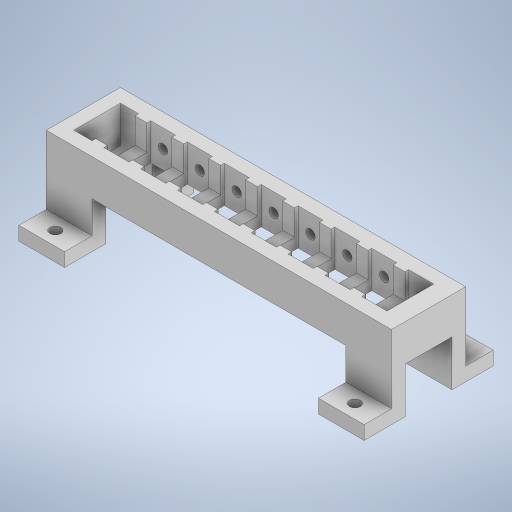
# Autodesk Inventor part: LatchBank
Saved by Autodesk Inventor 2024 (Build 280153000, 153)
## iProperties
Created: 2023-10-31
Part Number: LatchBank
Material: Generic
Document SubType Name: Modeling
Designer: gcter
Density: 1 g/cm^3
Appearance: Default
Author: gcter
Autodesk Inventor part; units mm, degrees
ref_plane "YZ Plane" through (0, 0, 0) normal (1, 0, 0) x (0, 1, 0)
ref_plane "XZ Plane" through (0, 0, 0) normal (0, 1, 0) x (-1, 0, 0)
ref_plane "XY Plane" through (0, 0, 0) normal (0, 0, 1) x (1, 0, 0)
sketch "Sketch1" plane through (0, 0, 0) normal (0, 1, 0) x (-1, 0, 0)
  line L0 (0, 0) -> (-5.08, 0)
  line L1 (-3.81, -3.81) -> (-3.81, -16.764)
  line L2 (-3.81, -20.574) -> (0, -20.574)
  line L3 (0, -20.574) -> (0, 0)
  line L4 (-3.81, -20.574) -> (-8.89, -20.574)
  line L5 (-8.89, -16.764) -> (-3.81, -16.764)
  line L6 (-3.81, -3.81) -> (-8.89, -3.81)
  line L7 (-5.08, 0) -> (-8.89, 0)
  line L8 (-8.89, -20.574) -> (-8.89, -16.764)
  line L9 (-8.89, -3.81) -> (-8.89, 0)
  point P0 (-1.905, -20.574)
  point P1 (-2.54, 0)
  point P2 (-3.81, -9.144)
  dimension "d1" = 20.574
  dimension "d4" = 3.81
  dimension "d7" = 3.81
  dimension "d28" = 3.81
  dimension "d47" = 5.08
  constraints: 20 end point, 4 horizontal, 3 parallel, 2 collinear, 2 midpoint, 2 point on line, 1 perpendicular
  measures "d1" distance from line of point (-2.54, 0) L2
  measures "d4" distance between parallel lines of L5 L4
  measures "d7" distance between parallel lines of L3 L1
  measures "d28" distance between parallel lines of L7 L6
  measures "d47" distance between parallel lines of L8 L1
extrude "Extrusion1" add sketch "Sketch1" along normal blind 10.16
sketch "Sketch6" plane through (0, 0, 0) normal (0, -1, 0) x (1, 0, 0)
  line L0 (13.975, -20.574) -> (8.89, -20.574)
  line L1 (8.89, -20.574) -> (8.89, -15.748)
  line L2 (8.89, -15.748) -> (12.192, -15.748)
  line L3 (12.192, -15.748) -> (12.192, -16.764)
  line L4 (8.89, -20.574) -> (0, -20.574) projected
  line L5 (8.89, -16.764) -> (8.89, -20.574) projected
  line L6 (12.192, -4.826) -> (8.89, -4.826)
  line L7 (8.89, -4.826) -> (8.89, 0)
  line L8 (8.89, 0) -> (13.4866, 0)
  line L9 (12.192, -3.81) -> (12.192, -4.826)
  line L10 (0, 0) -> (8.89, 0) projected
  line L11 (8.89, 0) -> (8.89, -3.81) projected
  line L12 (19.1262, -20.574) -> (13.975, -20.574)
  line L13 (12.192, -16.764) -> (19.1262, -16.764)
  line L14 (19.1262, -16.764) -> (19.1262, -20.574)
  line L15 (19.1262, -3.81) -> (12.192, -3.81)
  line L16 (13.4866, 0) -> (19.1262, 0)
  line L17 (19.1262, 0) -> (19.1262, -3.81)
  line L18 (3.81, -16.764) -> (8.89, -16.764) projected
  line L19 (8.89, -3.81) -> (3.81, -3.81) projected
  dimension "d48" = 1.016
  dimension "d49" = 1.016
  dimension "d50" = 3.302
  dimension "d51" = 6.9342
  constraints: 28 end point, 10 collinear, 6 parallel, 4 horizontal, 2 perpendicular
  measures "d48" distance between parallel lines of L15 L6
  measures "d49" distance between parallel lines of L2 L13
  measures "d50" distance between parallel lines of L1 L3
  measures "d51" distance between parallel lines of L3 L14
extrude "Extrusion5" add sketch "Sketch6" against normal up to surface (10.16 mm away)
sketch "Sketch7" plane through (12.192, 0, -16.764) normal (0, 0, 1) x (1, 0, 0)
  line L0 (6.9342, 10.16) -> (0, 10.16) construction
  line L1 (0, 0) -> (0, 10.16) construction
  line L2 (6.9342, 0) -> (6.9342, 10.16) construction
  line L3 (6.9342, 0) -> (0, 0) construction
  line L4 (0, 10.16) -> (6.9342, 0) construction
  line L5 (6.9342, 10.16) -> (0, 0) construction
  circle A0 centre (3.4671, 5.08) radius 1.3
  point P0 (-12.192, 0)
  dimension "d54" = 2.6
  constraints: 4 end point, 1 centre point, 1 midpoint
  measures "d54" diameter of A0
extrude "Extrusion6" cut sketch "Sketch7" against normal up to surface (3.81 mm away)
sketch "Sketch8" plane through (0, 0, 0) normal (0, -1, 0) x (1, 0, 0)
  line L0 (8.89, -3.81) -> (8.89, -4.826) construction
  line L1 (12.192, -4.826) -> (12.192, -3.81) construction
  line L2 (8.89, -15.748) -> (8.89, -16.764) construction
  line L3 (12.192, -16.764) -> (12.192, -15.748) construction
  line L4 (8.89, -4.826) -> (12.192, -4.826) construction
  line L5 (12.192, -15.748) -> (8.89, -15.748) construction
  line L6 (8.89, -4.826) -> (12.192, -4.826)
  line L7 (12.192, -4.826) -> (12.192, -15.748)
  line L8 (12.192, -15.748) -> (8.89, -15.748)
  line L9 (8.89, -15.748) -> (8.89, -4.826)
  point P0 (0, 0)
  constraints: 8 end point, 4 collinear, 2 parallel, 1 horizontal, 1 perpendicular
extrude "Extrusion7" add sketch "Sketch8" against normal blind 3.048
pattern_linear "Rectangular Pattern3" count 8 spacing 10.2362 along (1, 0, 0) of "Extrusion6", "Extrusion5", "Extrusion7"
sketch "Sketch9" plane through (90.7796, 0, -16.764) normal (1, 0, 0) x (0, 0, -1)
  line L0 (3.81, 0) -> (3.81, 10.16) construction
  line L1 (3.81, 10.16) -> (0, 10.16) construction
  line L2 (3.81, 0) -> (0, 0) construction
  line L3 (-12.954, 10.16) -> (-16.764, 10.16) construction
  line L4 (-16.764, 0) -> (-16.764, 10.16) construction
  line L5 (-12.954, 0) -> (-16.764, 0) construction
  line L6 (3.81, 10.16) -> (-16.764, 10.16)
  line L7 (-16.764, 10.16) -> (-16.764, 0)
  line L8 (-16.764, 0) -> (3.81, 0)
  line L9 (3.81, 0) -> (3.81, 10.16)
  constraints: 8 end point, 4 collinear, 2 parallel, 1 horizontal, 1 perpendicular
extrude "Extrusion8" add sketch "Sketch9" along normal blind 5.08
sketch "Sketch10" plane through (0, 0, 0) normal (0, -1, 0) x (1, 0, 0)
  line L0 (0, -20.574) -> (0, 0) construction
  line L1 (0, 0) -> (95.8596, 0) construction
  line L2 (95.8596, 0) -> (95.8596, -20.574) construction
  line L3 (0, -20.574) -> (95.8596, -20.574) construction
  line L4 (3.81, -16.764) -> (8.89, -16.764) construction
  line L5 (8.89, -3.81) -> (3.81, -3.81) construction
  line L6 (83.8454, -3.81) -> (90.7796, -3.81) construction
  line L7 (90.7796, -16.764) -> (83.8454, -16.764) construction
  line L8 (0, 0) -> (12.7, 0)
  line L9 (12.7, 0) -> (12.7, -3.81)
  line L10 (12.7, -3.81) -> (0, -3.81)
  line L11 (0, -3.81) -> (0, 0)
  line L12 (0, -16.764) -> (12.7, -16.764)
  line L13 (12.7, -16.764) -> (12.7, -20.574)
  line L14 (12.7, -20.574) -> (0, -20.574)
  line L15 (0, -20.574) -> (0, -16.764)
  line L16 (83.1596, 0) -> (95.8596, 0)
  line L17 (95.8596, 0) -> (95.8596, -3.81)
  line L18 (95.8596, -3.81) -> (83.1596, -3.81)
  line L19 (83.1596, -3.81) -> (83.1596, 0)
  line L20 (83.1596, -16.764) -> (95.8596, -16.764)
  line L21 (95.8596, -16.764) -> (95.8596, -20.574)
  line L22 (95.8596, -20.574) -> (83.1596, -20.574)
  line L23 (83.1596, -20.574) -> (83.1596, -16.764)
  dimension "d64" = 12.7
  dimension "d65" = 12.7
  dimension "d66" = 12.7
  dimension "d67" = 12.7
  constraints: 32 end point, 11 collinear, 8 parallel, 4 horizontal, 4 perpendicular, 1 point on line
  measures "d64" distance between parallel lines of L2 L19
  measures "d65" distance between parallel lines of L23 L2
  measures "d66" distance between parallel lines of L0 L9
  measures "d67" distance between parallel lines of L13 L0
extrude "Extrusion9" add sketch "Sketch10" along normal blind 12.7
sketch "Sketch11" plane through (95.8596, 10.16, -20.574) normal (0, 0, -1) x (-1, 0, 0)
  point P0 (95.8596, -10.16)
sketch "Sketch12" plane through (0, -12.7, 0) normal (0, -1, 0) x (1, 0, 0)
  line L0 (83.1596, -16.764) -> (83.1596, -20.574) construction
  line L1 (83.1596, -20.574) -> (95.8596, -20.574) construction
  line L2 (95.8596, -20.574) -> (95.8596, -16.764) construction
  line L3 (95.8596, -3.81) -> (95.8596, 0) construction
  line L4 (95.8596, 0) -> (83.1596, 0) construction
  line L5 (83.1596, 0) -> (83.1596, -3.81) construction
  line L6 (12.7, -20.574) -> (12.7, -16.764) construction
  line L7 (0, -20.574) -> (12.7, -20.574) construction
  line L8 (0, -16.764) -> (0, -20.574) construction
  line L9 (0, 0) -> (0, -3.81) construction
  line L10 (12.7, 0) -> (0, 0) construction
  line L11 (12.7, -3.81) -> (12.7, 0) construction
  line L12 (95.8596, 0) -> (83.1596, 0)
  line L13 (83.1596, 0) -> (83.1596, 7.62)
  line L14 (83.1596, 7.62) -> (95.8596, 7.62)
  line L15 (95.8596, 7.62) -> (95.8596, 0)
  line L16 (95.8596, -28.194) -> (83.1596, -28.194)
  line L17 (83.1596, -28.194) -> (83.1596, -20.574)
  line L18 (83.1596, -20.574) -> (95.8596, -20.574)
  line L19 (95.8596, -20.574) -> (95.8596, -28.194)
  line L20 (12.7, -28.194) -> (0, -28.194)
  line L21 (0, -28.194) -> (0, -20.574)
  line L22 (0, -20.574) -> (12.7, -20.574)
  line L23 (12.7, -20.574) -> (12.7, -28.194)
  line L24 (12.7, 0) -> (0, 0)
  line L25 (0, 0) -> (0, 7.62)
  line L26 (0, 7.62) -> (12.7, 7.62)
  line L27 (12.7, 7.62) -> (12.7, 0)
  point P0 (6.35, 7.62)
  dimension "d70" = 7.62
  dimension "d71" = 7.62
  dimension "d72" = 7.62
  dimension "d73" = 7.62
  constraints: 32 end point, 11 collinear, 8 parallel, 4 horizontal, 4 perpendicular, 1 midpoint, 1 point on line
  measures "d70" distance between parallel lines of L1 L16
  measures "d71" distance between parallel lines of L4 L14
  measures "d72" distance between parallel lines of L7 L20
  measures "d73" distance from line of point (6.35, 7.62) L10
extrude "Extrusion10" add sketch "Sketch12" against normal blind 3.81
sketch "Sketch13" plane through (0, -8.89, 0) normal (0, 1, 0) x (1, 0, 0)
  line L0 (83.1596, 28.194) -> (83.1596, 20.574) construction
  line L1 (95.8596, 28.194) -> (83.1596, 28.194) construction
  line L2 (95.8596, 20.574) -> (95.8596, 28.194) construction
  line L3 (12.7, 20.574) -> (12.7, 28.194) construction
  line L4 (12.7, 28.194) -> (0, 28.194) construction
  line L5 (0, 28.194) -> (0, 20.574) construction
  line L6 (0, 0) -> (0, -7.62) construction
  line L7 (0, -7.62) -> (12.7, -7.62) construction
  line L8 (12.7, -7.62) -> (12.7, 0) construction
  line L9 (83.1596, 0) -> (83.1596, -7.62) construction
  line L10 (83.1596, -7.62) -> (95.8596, -7.62) construction
  line L11 (95.8596, -7.62) -> (95.8596, 0) construction
  line L12 (95.8596, -7.62) -> (83.1596, 0) construction
  line L13 (0, 0) -> (95.8596, 0) construction
  line L14 (83.1596, -7.62) -> (95.8596, 0) construction
  line L15 (95.8596, 20.574) -> (83.1596, 20.574) construction
  line L16 (95.8596, 20.574) -> (83.1596, 28.194) construction
  line L17 (83.1596, 20.574) -> (95.8596, 28.194) construction
  line L18 (12.7, 28.194) -> (0, 20.574) construction
  line L19 (12.7, 20.574) -> (0, 28.194) construction
  line L20 (0, -7.62) -> (12.7, 0) construction
  line L21 (12.7, -7.62) -> (0, 0) construction
  circle A0 centre (6.35, -3.81) radius 1.524
  circle A1 centre (89.5096, -3.81) radius 1.524
  circle A2 centre (6.35, 24.384) radius 1.524
  circle A3 centre (89.5096, 24.384) radius 1.524
  point P0 (6.35, -3.81)
  point P1 (89.5096, 24.384)
  dimension "d77" = 3.048
  dimension "d78" = 3.048
  dimension "d79" = 3.048
  dimension "d80" = 3.048
  constraints: 16 end point, 4 centre point, 4 coincident, 4 midpoint, 4 parallel
  measures "d77" diameter of A0
  measures "d78" diameter of A1
  measures "d79" diameter of A2
  measures "d80" diameter of A3
extrude "Extrusion11" cut sketch "Sketch13" against normal up to surface (3.81 mm away)
body "Solid1"
